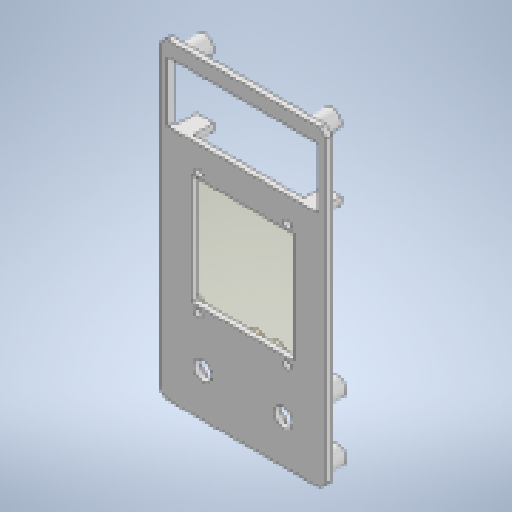
# Autodesk Inventor part: Housing Top
Saved by Autodesk Inventor 2023 (Build 270158000, 158)
## iProperties
Created: 2023-06-04
Part Number: Housing Top
Material: Generic
Document SubType Name: Modeling
Designer: jeffb
Density: 1 g/cm^3
Appearance: Default
Author: jeffb
Autodesk Inventor part; units mm, degrees
ref_plane "YZ Plane" through (0, 0, 0) normal (1, 0, 0) x (0, 1, 0)
ref_plane "XZ Plane" through (0, 0, 0) normal (0, 1, 0) x (-1, 0, 0)
ref_plane "XY Plane" through (0, 0, 0) normal (0, 0, 1) x (1, 0, 0)
ref_plane "Work Plane1" through (0, 0, 0) normal (0, 0, 1) x (1, 0, 0)
sketch "Sketch1" plane through (0, 0, 0) normal (0, 0, 1) x (1, 0, 0)
  line L0 (-17.027, -17.996) -> (16.773, -17.996) construction
  line L1 (16.773, -17.996) -> (16.773, 18.504) construction
  line L2 (16.773, 18.504) -> (-17.027, 18.504) construction
  line L3 (-17.027, 18.504) -> (-17.027, -17.996) construction
  line L4 (-13.557, 17.104) -> (13.303, 17.104) construction
  line L5 (13.303, 17.104) -> (13.303, -9.756) construction
  line L6 (13.303, -9.756) -> (-13.557, -9.756) construction
  line L7 (-13.557, -9.756) -> (-13.557, 17.104) construction
  line L8 (-17.652, -18.621) -> (17.398, -18.621)
  line L9 (17.398, -18.621) -> (17.398, 19.129)
  line L10 (17.398, 19.129) -> (-17.652, 19.129)
  line L11 (-17.652, 19.129) -> (-17.652, -18.621)
  circle A0 centre (15.24, 20.955) radius 1.25 construction
  circle A1 centre (-15.24, 20.955) radius 1.25 construction
  circle A2 centre (-15.24, -20.955) radius 1.25 construction
  circle A3 centre (15.24, -20.955) radius 1.25 construction
  circle A4 centre (-15.24, 20.955) radius 1.25
  circle A5 centre (15.24, 20.955) radius 1.25
  circle A6 centre (15.24, -20.955) radius 1.25
  circle A7 centre (-15.24, -20.955) radius 1.25
  circle A8 centre (-13.8215, -37.1488) radius 3 construction
  circle A9 centre (13.7785, -37.1488) radius 3 construction
  line L12 (-25.2, 30.13) -> (25.2, 30.13) construction
  line L13 (25.2, 30.13) -> (25.2, 49.53) construction
  line L14 (25.2, 49.53) -> (-25.2, 49.53) construction
  line L15 (-25.2, 49.53) -> (-25.2, 30.13) construction
  circle A10 centre (-13.8215, -37.1488) radius 3.175
  circle A11 centre (13.7785, -37.1488) radius 3.175
  line L16 (-25.825, 50.155) -> (25.825, 50.155)
  line L17 (25.825, 50.155) -> (25.825, 29.505)
  line L18 (25.825, 29.505) -> (-25.825, 29.505)
  line L19 (-25.825, 29.505) -> (-25.825, 50.155)
  line L20 (-26.2766, -51.835) -> (26.2766, -51.835) projected
  arc A12 (-28.5, -49.6116) -> (-26.2766, -51.835) centre (-23.5, -46.835) ccw projected
  line L21 (-28.5, 52.9416) -> (-28.5, -49.6116) projected
  arc A13 (-26.2766, 55.165) -> (-28.5, 52.9416) centre (-23.5, 50.165) ccw projected
  line L22 (26.2766, 55.165) -> (-26.2766, 55.165) projected
  arc A14 (28.5, 52.9416) -> (26.2766, 55.165) centre (23.5, 50.165) ccw projected
  line L23 (28.5, -49.6116) -> (28.5, 52.9416) projected
  arc A15 (26.2766, -51.835) -> (28.5, -49.6116) centre (23.5, -46.835) ccw projected
  arc A16 (30.5, 53.4186) -> (26.7536, 57.165) centre (23.5, 50.165) ccw projected
  line L24 (-26.7536, 57.165) -> (26.7536, 57.165) projected
  arc A17 (-26.7536, 57.165) -> (-30.5, 53.4186) centre (-23.5, 50.165) ccw projected
  line L25 (-30.5, -50.0886) -> (-30.5, 53.4186) projected
  arc A18 (-30.5, -50.0886) -> (-26.7536, -53.835) centre (-23.5, -46.835) ccw projected
  line L26 (26.7536, -53.835) -> (-26.7536, -53.835) projected
  arc A19 (26.7536, -53.835) -> (30.5, -50.0886) centre (23.5, -46.835) ccw projected
  line L27 (30.5, 53.4186) -> (30.5, -50.0886) projected
  point P0 (0, 0)
  dimension "d0" = 0.625
  dimension "d1" = 6.35
  dimension "d2" = 6.35
  dimension "d3" = 0.625
  constraints: 16 end point, 6 centre point, 6 coincident, 4 equal radius, 6 other
  measures "d0" distance between parallel lines of L3 L11
  measures "d1" diameter of A10
  measures "d2" diameter of A11
  measures "d3" distance between parallel lines of L14 L16
extrude "Extrusion1" add sketch "Sketch1" along normal blind 2 contours A12 L21 A13 L22 A14 L23 A15 L20
sketch "Sketch3" plane through (0, 0, 0) normal (0, 0, -1) x (-1, 0, 0)
  circle A0 centre (-21.844, 51.26) radius 1 construction
  circle A1 centre (21.846, 51.26) radius 1 construction
  circle A2 centre (-21.844, 28.4) radius 1 construction
  circle A3 centre (21.846, 28.4) radius 1 construction
  circle A4 centre (21.846, 51.26) radius 0.8509
  circle A5 centre (21.846, 28.4) radius 0.8509
  circle A6 centre (-21.844, 51.26) radius 0.8509
  circle A7 centre (-21.844, 28.4) radius 0.8509
  arc A8 (-28.5, -49.6116) -> (-26.2766, -51.835) centre (-23.5, -46.835) ccw
  line L0 (26.2766, -51.835) -> (-26.2766, -51.835)
  arc A9 (26.2766, -51.835) -> (28.5, -49.6116) centre (23.5, -46.835) ccw
  line L1 (28.5, 52.9416) -> (28.5, -49.6116)
  arc A10 (28.5, 52.9416) -> (26.2766, 55.165) centre (23.5, 50.165) ccw
  line L2 (-26.2766, 55.165) -> (26.2766, 55.165)
  arc A11 (-26.2766, 55.165) -> (-28.5, 52.9416) centre (-23.5, 50.165) ccw
  line L3 (-28.5, -49.6116) -> (-28.5, 52.9416)
  circle A12 centre (15.24, 20.955) radius 1.25
  circle A13 centre (-15.24, 20.955) radius 1.25
  circle A14 centre (-15.24, -20.955) radius 1.25
  circle A15 centre (15.24, -20.955) radius 1.25
  circle A16 centre (13.8215, -37.1488) radius 3.175
  circle A17 centre (-13.7785, -37.1488) radius 3.175
  line L4 (25.825, 50.155) -> (-25.825, 50.155)
  line L5 (25.825, 29.505) -> (25.825, 50.155)
  line L6 (-25.825, 29.505) -> (25.825, 29.505)
  line L7 (-25.825, 50.155) -> (-25.825, 29.505)
  line L8 (17.652, -18.621) -> (17.652, 19.129)
  line L9 (-17.398, -18.621) -> (17.652, -18.621)
  line L10 (-17.398, 19.129) -> (-17.398, -18.621)
  line L11 (17.652, 19.129) -> (-17.398, 19.129)
  circle A18 centre (21.846, 51.26) radius 3.175
  circle A19 centre (-21.844, 51.26) radius 3.175
  circle A20 centre (-21.844, 28.4) radius 3.175
  circle A21 centre (21.846, 28.4) radius 3.175
  point P0 (0, 0)
  point P1 (-24.8205, 29.505)
  point P2 (-18.8675, 29.505)
  point P3 (-18.8675, 50.155)
  point P4 (-24.8205, 50.155)
  point P5 (24.8225, 50.155)
  point P6 (18.8695, 50.155)
  point P7 (18.8695, 29.505)
  point P8 (24.8225, 29.505)
  dimension "d6" = 1.7018
  dimension "d7" = 6.35
  constraints: 24 end point, 18 centre point, 8 coincident, 8 point on circle, 6 equal radius
  measures "d6" diameter of A6
  measures "d7" diameter of A18
ref_plane "Work Plane2" through (-25.02, 26.495, -6.9) normal (0, 0, 1) x (1, 0, 0)
extrude "Extrusion2" add sketch "Sketch3" along normal up to surface (6.9 mm away) contours L4 A18 | A21 L6 | L4 A19 | A20 L6 picked at (24.2052, 51.5895) picked at (24.2052, 28.0705) picked at (-19.4848, 51.5895) picked at (-19.4848, 28.0705)
sketch "Sketch4" plane through (0, 0, 0) normal (0, 0, -1) x (-1, 0, 0)
  circle A0 centre (-23.96, -26.975) radius 1.25 construction
  circle A1 centre (-23.96, -47.295) radius 1.25 construction
  circle A2 centre (-3.64, -47.295) radius 1.25 construction
  circle A3 centre (-3.64, -26.975) radius 1.25 construction
  circle A4 centre (3.64, -26.975) radius 1.25 construction
  circle A5 centre (3.64, -47.295) radius 1.25 construction
  circle A6 centre (23.96, -47.295) radius 1.25 construction
  circle A7 centre (23.96, -26.975) radius 1.25 construction
  circle A8 centre (-23.96, -26.975) radius 3.175
  circle A9 centre (-23.96, -47.295) radius 3.175
  circle A10 centre (-3.64, -47.295) radius 3.175
  circle A11 centre (3.64, -47.295) radius 3.175
  circle A12 centre (23.96, -47.295) radius 3.175
  circle A13 centre (23.96, -26.975) radius 3.175
  circle A14 centre (3.64, -26.975) radius 3.175
  circle A15 centre (-3.64, -26.975) radius 3.175
  circle A16 centre (3.64, -47.295) radius 0.8509
  circle A17 centre (23.96, -47.295) radius 0.8509
  circle A18 centre (-23.96, -47.295) radius 0.8509
  circle A19 centre (-3.64, -47.295) radius 0.8509
  circle A20 centre (23.96, -26.975) radius 0.8509
  circle A21 centre (3.64, -26.975) radius 0.8509
  circle A22 centre (-3.64, -26.975) radius 0.8509
  circle A23 centre (-23.96, -26.975) radius 0.8509
  point P0 (0, 0)
  dimension "d10" = 6.35
  dimension "d11" = 6.35
  dimension "d12" = 6.35
  dimension "d13" = 6.35
  dimension "d14" = 6.35
  dimension "d15" = 6.35
  dimension "d16" = 6.35
  dimension "d17" = 6.35
  dimension "d18" = 1.7018
  dimension "d19" = 1.7018
  dimension "d20" = 1.7018
  dimension "d21" = 1.7018
  dimension "d22" = 1.7018
  dimension "d23" = 1.7018
  dimension "d24" = 1.7018
  dimension "d25" = 1.7018
  constraints: 16 centre point, 16 coincident
  measures "d10" diameter of A8
  measures "d11" diameter of A9
  measures "d12" diameter of A10
  measures "d13" diameter of A11
  measures "d14" diameter of A12
  measures "d15" diameter of A13
  measures "d16" diameter of A14
  measures "d17" diameter of A15
  measures "d18" diameter of A16
  measures "d19" diameter of A17
  measures "d20" diameter of A18
  measures "d21" diameter of A19
  measures "d22" diameter of A20
  measures "d23" diameter of A21
  measures "d24" diameter of A22
  measures "d25" diameter of A23
ref_plane "Work Plane3" through (-26.5, -49.835, -6.5) normal (0, 0, 1) x (1, 0, 0)
extrude "Extrusion3" add sketch "Sketch4" along normal up to surface (6.5 mm away)
body "Solid1"
